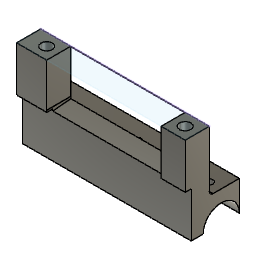
brake attachment v7 (Autodesk Fusion 360 design; units mm, degrees)
Autodesk Fusion 360 part; units mm, degrees
note: some values were not read from the file. Chosen so that the rebuilt part matches the saved one: which face or edge a step refers to. Set by a fixed rule: which sketch regions a step uses.
sketch "Sketch2" plane through (0, 0, 0) normal (1, 0, 0) x (0, 1, 0)
  line L0 (0, 0) -> (28.575, 0)
  line L1 (28.575, 0) -> (28.575, 12.7)
  line L2 (28.575, 12.7) -> (0, 12.7)
  line L3 (0, 12.7) -> (0, 0)
  line L4 (0, 0) -> (15.875, 0)
  line L5 (15.875, 0) -> (19.05, 0)
  circle A0 centre (19.05, 0) radius 9.525
  line L6 (28.575, 0) -> (19.05, 0)
  dimension "d1" = 28.575
  dimension "d2" = 12.7
  dimension "d3" = 15.875
  dimension "d5" = 19.05
  dimension "d37" = 9.525
  constraint horizontal L0
  constraint vertical L1
  constraint horizontal L2
  constraint vertical L3
  constraint coincident L0.start L3.end
  constraint perpendicular L3 L4
  constraint parallel L0 L5
  constraint coincident L5.end A0.centre
  constraint perpendicular L1 L6
  measures "d1" distance of L0.start L0.end
  measures "d2" distance of L0.start L2.end
  measures "d3" distance of L0.start L4.end
  measures "d5" diameter of A0
  measures "d37" distance of L0.end L5.end
extrude "Extrude1" add sketch "Sketch2" along normal blind 88.9 contours L0 L1 L2 L3 L4 A0
sketch "Sketch3" plane through (88.9, 0, 0) normal (1, 0, 0) x (0, 1, 0)
  line L0 (28.575, 12.7) -> (0, 12.7)
  line L1 (0, 12.7) -> (0, 0)
  line L2 (0, 0) -> (9.525, 0)
  arc A0 (28.575, 0) -> (9.525, 0) centre (19.05, 0) ccw
  line L3 (28.575, 0) -> (28.575, 12.7)
  line L4 (0, 0) -> (15.875, 0)
  line L5 (15.875, 0) -> (15.875, 12.7)
  line L6 (0, 12.7) -> (0, 47.625)
  line L7 (0, 47.625) -> (12.7, 47.625)
  line L8 (0, 12.7) -> (15.875, 12.7)
  line L9 (12.7, 47.625) -> (12.7, 12.7)
  line L10 (28.575, 12.7) -> (12.7, 12.7)
  line L11 (12.7, 12.7) -> (12.7, 15.875)
  line L12 (12.7, 15.875) -> (28.575, 15.875)
  line L13 (28.575, 15.875) -> (28.575, 12.7)
  dimension "d8" = 15.875
  dimension "d9" = 12.7
  dimension "d10" = 34.925
  dimension "d11" = 12.7
  dimension "d54" = 3.175
  constraint coincident L1.end L2.start
  constraint coincident L2.end L4.end
  constraint perpendicular L2 L5
  constraint coincident L0.end L1.start
  constraint perpendicular L0 L6
  constraint perpendicular L6 L7
  constraint perpendicular L5 L8
  constraint horizontal L10
  constraint vertical L11
  constraint horizontal L12
  constraint vertical L13
  measures "d8" distance of L1.end L4.end
  measures "d9" distance of L4.end L5.end
  measures "d10" distance of L0.end L6.end
  measures "d11" distance of L6.end L7.end
  measures "d54" distance of L0.start L12.end
extrude "Extrude2" add sketch "Sketch3" against normal blind 88.9 contours L0 L6 L7 L8 L9 L11
sketch "Sketch4" plane through (0, 0, 47.625) normal (0, 0, 1) x (-1, 0, 0)
  line L0 (-88.9, 0) -> (-88.9, -12.7)
  line L1 (0, -12.7) -> (0, 0)
  line L2 (0, 0) -> (-88.9, 0)
  line L3 (-88.9, -12.7) -> (0, -12.7)
sketch "Sketch5" plane through (0, 0, 47.625) normal (0, 0, 1) x (-1, 0, 0)
  line L0 (0, 0) -> (-101.6, 0)
  line L1 (0, 0) -> (-9.525, 0)
  line L2 (-101.6, 0) -> (-95.25, 0)
  line L3 (0, 0) -> (0, -12.7)
  line L4 (0, 0) -> (0, -9.525)
  circle A0 centre (-9.5229, -6.3508) radius 2.9997
  circle A1 centre (-82.5479, -6.3355) radius 2.9997
  circle A2 centre (-6.35, -19.05) radius 1.5113
  circle A3 centre (-82.546, -19.0347) radius 1.5113
  circle A4 centre (-44.45, -19.0424) radius 1.5113
  line L5 (-6.35, -19.05) -> (-6.3489, -19.05)
  line L6 (-6.3489, -19.05) -> (-44.45, -19.0424)
  line L7 (-44.45, -19.0424) -> (-82.546, -19.0347)
  dimension "d16" = 101.6
  dimension "d17" = 9.525
  dimension "d19" = 9.525
  dimension "d20" = 5.9995
  dimension "d22" = 5.9995
  dimension "d25" = 3.0226
  dimension "d26" = 3.0226
  dimension "d27" = 38.1
  dimension "d28" = 3.0226
  constraint coincident L0.start L1.start
  constraint horizontal L0
  constraint parallel L0 L1
  constraint parallel L0 L2
  constraint perpendicular L1 L3
  constraint perpendicular L0 L4
  constraint coincident A2.centre L5.start
  constraint coincident A4.centre L6.end
  constraint coincident A3.centre L7.end
  measures "d16" distance of L0.start L0.end
  measures "d17" distance of L0.start L1.end
  measures "d19" distance of L0.start L4.end
  measures "d20" diameter of A0
  measures "d22" diameter of A1
  measures "d25" diameter of A2
  measures "d26" diameter of A3
  measures "d27" distance of A2.centre A4.centre
  measures "d28" diameter of A4
hole "Hole2" at (9.5229, 6.3508, 47.625) at (82.5479, 6.3355, 47.625) direction (0, 0, -1) diameter 5.9995 depth 19.05 tip angle 180
sketch "Sketch6" plane through (0, 0, 0) normal (-1, 0, 0) x (0, -1, 0)
  line L0 (-12.7, 12.7) -> (-28.575, 12.7)
  line L1 (-28.575, 12.7) -> (-28.575, 0)
  arc A0 (-9.525, 0) -> (-28.575, 0) centre (-19.05, 0) ccw
  line L2 (-9.525, 0) -> (0, 0)
  line L3 (0, 0) -> (0, 47.625)
  line L4 (0, 47.625) -> (-12.7, 47.625)
  line L5 (0, 47.625) -> (0, 0)
  line L6 (0, 0) -> (0, 47.625)
  line L7 (0, 47.625) -> (0, 0)
  line L8 (-12.7, 47.625) -> (-12.7, 0)
  line L9 (-28.575, 0) -> (0, 0)
  line L10 (0, 0) -> (-6.35, 0)
  line L11 (0, 0) -> (-3.175, 0)
  line L12 (-3.175, 0) -> (-3.175, 23.8125)
  line L13 (-3.175, 23.8125) -> (0, 23.8125)
  line L14 (0, 23.8125) -> (0, 0)
  line L15 (-19.05, 0) -> (0, 0)
  line L16 (-12.7, 47.625) -> (-12.7, 12.7)
  dimension "d38" = 6.35
  dimension "d39" = 3.175
  dimension "d40" = 23.8125
  constraint coincident L3.end L4.start
  constraint coincident L2.end L3.start
  constraint coincident L4.end L8.start
  constraint perpendicular L0 L8
  constraint coincident L1.end A0.end
  constraint perpendicular L3 L10
  constraint horizontal L11
  constraint vertical L12
  constraint horizontal L13
  constraint vertical L14
  constraint coincident A0.centre L15.start
  measures "d38" distance of L2.end L10.end
  measures "d39" distance of L2.end L11.end
  measures "d40" distance of L2.end L13.end
extrude "Extrude3" cut sketch "Sketch6" against normal blind 101.6 contours L2 L3 L5 L6 L7 L9 L10 L11 L12 L13 L14 L15
sketch "Sketch8" plane through (0, 16.89, 1.5355) normal (0, 0.995893, 0.090536) x (-1, 0, 0)
  line L0 (-88.9, 46.2796) -> (-88.9, 11.2106)
  line L1 (-88.9, 11.2106) -> (0, 11.2106)
  line L2 (0, 11.2106) -> (0, 46.2796)
  line L3 (0, 46.2796) -> (-88.9, 46.2796)
  line L4 (0, 0) -> (-88.9, 0)
  line L5 (-6.2953, 46.2796) -> (0, 46.2796)
  line L6 (-76.2265, 46.2796) -> (-15.9015, 46.2796)
  line L7 (-15.9015, 46.2796) -> (-15.9015, 22.4671)
  line L8 (-15.9015, 22.4671) -> (-76.2265, 22.4671)
  line L9 (-76.2265, 22.4671) -> (-76.2265, 46.2796)
  dimension "d43" = 60.325
  dimension "d44" = 23.8125
  constraint coincident L4.start origin
  constraint horizontal L4
  constraint coincident L3 L5.start
  constraint coincident L2.end L3.start
  constraint horizontal L6
  constraint vertical L7
  constraint horizontal L8
  constraint vertical L9
  constraint coincident L3 L6.start
  measures "d43" distance of L6.start L6.end
  measures "d44" distance of L6.start L8.end
sketch "Sketch9" plane through (0, 0, 47.625) normal (0, 0, 1) x (-1, 0, 0)
  line L0 (-15.8359, -12.5046) -> (-76.2, -12.5046)
  line L1 (-76.2, -12.5046) -> (-76.2, 0)
  line L2 (-76.2, 0) -> (-15.8359, 0)
  line L3 (-15.8359, 0) -> (-15.8359, -12.5046)
  constraint horizontal L0
  constraint vertical L1
  constraint horizontal L2
  constraint vertical L3
extrude "Extrude5" cut sketch "Sketch9" against normal blind 22.86
extrude "Extrude6" cut sketch "Sketch8" against normal blind 50.8 contours L3 L6 L7 L8 L9
extrude "Extrude7" add sketch "Sketch3" against normal blind 88.9 contours L0 L8 L9 L10 L11 L12 L13
hole "Hole1" at (6.35, 19.05, 47.625) at (82.546, 19.0347, 47.625) at (44.45, 19.0424, 47.625) direction (0, 0, -1) diameter 3.9878 depth 50.8 tip angle 118
fillet "Fillet2" radius 1.905 1 edges at (44.45, 12.7, 15.875)
